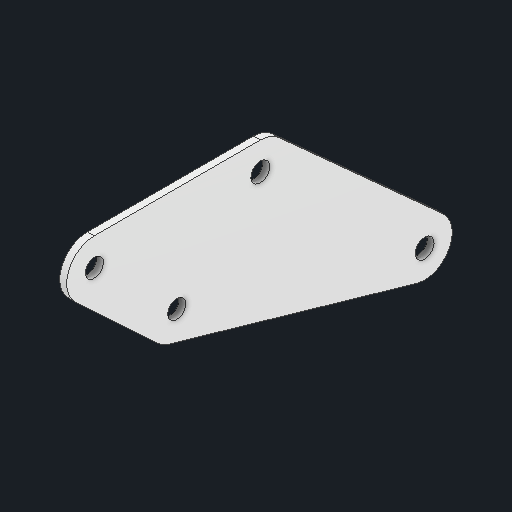
# Autodesk Inventor part: Gearbox
Saved by Autodesk Inventor 2025 (Build 290162000, 162)
## iProperties
Created: 2024-12-30
Part Number: Gearbox
Material: Acetal Resin, White
Document SubType Name: Modeling
Designer: Averey Ku
Density: 1.425 g/cm^3
Appearance: Smooth - White
Author: Averey Ku
Autodesk Inventor part; units mm, degrees
ref_plane "YZ Plane" through (0, 0, 0) normal (1, 0, 0) x (0, 1, 0)
ref_plane "XZ Plane" through (0, 0, 0) normal (0, 1, 0) x (-1, 0, 0)
ref_plane "XY Plane" through (0, 0, 0) normal (0, 0, 1) x (1, 0, 0)
sketch "main" plane through (0, 0, 0) normal (0, 0, 1) x (1, 0, 0)
  circle A0 centre (-3.3709, 14.5159) radius 2.0955
  arc A1 (-8.014, 18.8477) -> (-9.4735, 16.2713) centre (-3.3709, 14.5159) ccw
  line L0 (20.6421, 33.4478) -> (20.6421, -4.6562)
  line L1 (9.6491, 37.7797) -> (-8.014, 18.8477)
  arc A2 (20.6421, 33.4478) -> (9.6491, 37.7797) centre (14.2921, 33.4478) ccw
  circle A3 centre (14.2921, 33.4478) radius 2.0955
  circle A4 centre (14.2921, -4.6562) radius 2.1844
  arc A5 (18.9589, -8.9624) -> (20.6421, -4.6562) centre (14.2921, -4.6562) ccw
  line L2 (19.0546, -8.8563) -> (-15.0207, -46.629)
  circle A6 centre (-19.7356, -42.3756) radius 2.1844
  arc A7 (-25.8382, -40.6202) -> (-15.0207, -46.629) centre (-19.7356, -42.3756) ccw
  line L3 (-9.4735, 16.2713) -> (-25.8382, -40.6202)
  point P0 (2.8965, 2.4647)
  point P1 (16.3369, 32.8456)
  dimension "d1" = 4.191
  dimension "d2" = 12.7
  dimension "d3" = 12.7
  dimension "d4" = 12.7
  dimension "d5" = 12.7
  dimension "d6" = 4.191
  measures "d1" diameter of A3
  measures "d2" diameter of A2
  measures "d3" diameter of A7
  measures "d4" diameter of A5
  measures "d5" diameter of A1
  measures "d6" diameter of A0
sketch "Sketch1" plane through (0, 0, 0) normal (1, 0, 0) x (0, 1, 0)
  circle A0 centre (-17.663, -18.932) radius 2.0955
  arc A1 (-22.3061, -14.6001) -> (-23.7656, -17.1766) centre (-17.663, -18.932) ccw
  line L0 (6.35, 0) -> (6.35, -38.104)
  line L1 (-4.643, 4.3318) -> (-22.3061, -14.6001)
  arc A2 (6.35, 0) -> (-4.643, 4.3318) centre (0, 0) ccw
  circle A3 centre (0, 0) radius 2.0955
  circle A4 centre (0, -38.104) radius 2.1844
  arc A5 (4.6668, -42.4102) -> (6.35, -38.104) centre (0, -38.104) ccw
  line L2 (4.7625, -42.3042) -> (-29.3128, -80.0769)
  circle A6 centre (-34.0277, -75.8234) radius 2.1844
  arc A7 (-40.1303, -74.0681) -> (-29.3128, -80.0769) centre (-34.0277, -75.8234) ccw
  line L3 (-23.7656, -17.1766) -> (-40.1303, -74.0681)
extrude "Extrusion1" add sketch "Sketch1" along normal blind 1.5875
body "Solid1"
